Autodesk Fusion 360 part; units mm, degrees
(part 2 of 2)
  spline S76 degree 3 poles (-2.9132, -32.2574) (-2.9111, -32.1274) (-2.9075, -31.9972) (-2.9143, -31.8673) knots 0.000001 0.000001 0.000001 0.000001 1 1 1 1
  line L299 (-5.3918, -31.3025) -> (-5.3918, -30.7233)
  spline S77 degree 3 poles (3.2504, -31.7458) (3.2427, -31.2495) (3.2469, -30.7533) (3.249, -30.2573) knots 0 0 0 0 1 1 1 1
  spline S78 degree 3 poles (0.6248, -32.344) (0.4977, -32.344) (0.3707, -32.3426) (0.2432, -32.3447) knots 0.000001 0.000001 0.000001 0.000001 1 1 1 1
  line L300 (-9.9932, -29.679) -> (-9.9932, -31.7523)
  line L301 (-10.3578, -35.4986) -> (-10.0851, -35.4986)
  line L302 (3.8488, -30.2579) -> (3.8488, -31.7442)
  line L303 (-3.3074, -29.6804) -> (-3.3074, -32.3358)
  spline S79 degree 3 poles (-11.6128, -31.7979) (-11.6121, -31.7822) (-11.5583, -31.7551) (-11.5287, -31.7548) knots 0.000023 0.000023 0.000023 0.000023 1 1 1 1
  line L304 (2.2703, -31.4488) -> (2.2703, -29.6811)
  line L305 (-8.2179, -31.1386) -> (-8.2179, -31.7452)
  spline S80 degree 3 poles (3.249, -30.2573) (3.2504, -29.8676) (3.5651, -29.651) (3.862, -29.6709) knots 0 0 0 0 1 1 1 1
  line L306 (-6.7175, -30.5364) -> (-6.7175, -29.6794)
  line L307 (-8.2179, -31.7452) -> (-6.7246, -31.7452)
  line L308 (-9.9932, -31.7523) -> (-9.8717, -31.7523)
  spline S81 degree 3 poles (0.8918, -30.7238) (0.8571, -30.6827) (0.8217, -30.6427) (0.7622, -30.6077) (0.7622, -30.6076) (0.7621, -30.6076) (0.7621, -30.6076) knots 0 0 0 0 1 1 1 1.000845 1.000845 1.000845 1.000845
  spline S82 degree 3 poles (-0.9957, -31.7527) (-0.8318, -31.7527) (-0.8194, -31.7402) (-0.819, -31.5777) knots 0 0 0 0 1 1 1 1
  spline S83 degree 3 poles (2.1795, -31.3466) (2.2021, -31.3735) (2.2265, -31.3994) (2.2701, -31.4486) (2.2701, -31.4486) (2.2702, -31.4487) (2.2703, -31.4488) knots 0.000001 0.000001 0.000001 0.000001 1 1 1 1.001339 1.001339 1.001339 1.001339
  spline S84 degree 3 poles (-8.2309, -30.5512) (-7.7601, -30.5491) (-7.2897, -30.5459) (-6.8189, -30.5427) knots 0 0 0 0 1 1 1 1
  spline S85 degree 3 poles (-11.6167, -32.3309) (-11.6167, -32.1568) (-11.6188, -31.9773) (-11.6128, -31.7979) knots 0.000143 0.000143 0.000143 0.000143 1 1 1 1
  line L309 (-5.7649, -32.3358) -> (-5.7649, -31.7594)
  line L310 (-5.7639, -30.2551) -> (-5.7639, -29.6804)
  spline S86 degree 3 poles (-10.6833, -31.7527) (-10.6472, -31.7527) (-10.6111, -31.7495) (-10.5669, -31.747) (-10.5668, -31.747) (-10.5668, -31.747) (-10.5668, -31.747) knots 0.000001 0.000001 0.000001 0.000001 1 1 1 1.000711 1.000711 1.000711 1.000711
  line L311 (-6.7246, -31.1386) -> (-8.2179, -31.1386)
  spline S87 degree 3 poles (2.846, -32.3433) (2.6556, -32.3433) (2.4684, -32.3457) (2.2808, -32.3404) knots 0.000175 0.000175 0.000175 0.000175 1 1 1 1
  spline S88 degree 3 poles (-6.2574, -32.3358) (-6.907, -32.3358) (-7.5566, -32.3362) (-8.2061, -32.3358) knots 0 0 0 0 1 1 1 1
  spline S89 degree 3 poles (0.1693, -32.2743) (0.1711, -31.4188) (0.1715, -30.5632) (0.1725, -29.7076) knots 0 0 0 0 1 1 1 1
  spline S90 degree 3 poles (0.1845, -29.6744) (0.3647, -29.6744) (0.5431, -29.6705) (0.7211, -29.6776) knots 0.000128 0.000128 0.000128 0.000128 1 1 1 1
  spline S91 degree 3 poles (-0.8212, -29.6744) (-0.4737, -29.6744) (-0.2415, -29.9051) (-0.2408, -30.2531) knots 0 0 0 0 1 1 1 1
  line L312 (-6.7246, -31.7452) -> (-6.7246, -31.1386)
  spline S92 degree 3 poles (0.2432, -32.3447) (0.1916, -32.3454) (0.169, -32.3285) (0.1693, -32.2743) knots 0.000002 0.000002 0.000002 0.000002 1 1 1 1
  line L313 (6.3064, -30.2505) -> (6.3064, -29.6793)
  line L314 (-5.7649, -31.7594) -> (-3.8959, -31.7594)
  spline S93 degree 3 poles (-8.2061, -32.3358) (-8.5827, -32.3358) (-8.8163, -32.1023) (-8.8167, -31.7271) knots 0 0 0 0 1 1 1 1
  spline S94 degree 3 poles (-5.5311, -34.2712) (-5.5042, -34.6089) (-5.6574, -34.7776) (-5.9909, -34.7776) knots 0 0 0 0 1 1 1 1
  line L315 (-3.8959, -31.3025) -> (-5.3918, -31.3025)
  line L316 (-3.8959, -31.7594) -> (-3.8959, -31.3025)
  spline S95 degree 3 poles (3.862, -29.6709) (4.1049, -29.6868) (4.3498, -29.674) (4.5937, -29.674) knots 0 0 0 0 1 1 1 1
  line L317 (-3.8959, -30.2551) -> (-5.7639, -30.2551)
  spline S96 degree 3 poles (-11.707, -34.2199) (-11.6772, -33.5339) (-11.1336, -33.0249) (-10.4363, -33.0235) knots 0 0 0 0 1 1 1 1
  line L318 (-3.8959, -30.7233) -> (-3.8959, -30.2551)
  spline S97 degree 3 poles (-4.4917, -39.2977) (-4.5365, -39.296) (-4.612, -39.1654) (-4.6134, -39.0936) knots 0 0 0 0 1 1 1 1
  line L319 (-10.3578, -34.3815) -> (-10.3578, -35.4986)
  line L320 (-6.5701, -36.8485) -> (-10.1266, -36.8485)
  spline S98 degree 3 poles (-4.6191, -37.5707) (-4.6191, -36.5314) (-4.6223, -35.4917) (-4.618, -34.4524) knots 0 0 0 0 1 1 1 1
  line L321 (-6.5701, -35.8185) -> (-6.5701, -36.8485)
  line L322 (-2.7841, -30.2505) -> (-2.9061, -30.2505)
  line L323 (-0.819, -31.5777) -> (-0.819, -30.4279)
  line L324 (-5.3918, -30.7233) -> (-3.8959, -30.7233)
  spline S99 degree 3 poles (-6.6217, -34.7812) (-6.8333, -34.7978) (-6.9271, -34.7275) (-6.8956, -34.5116) knots 0 0 0 0 1 1 1 1
  line L325 (-10.1266, -37.9379) -> (-6.9307, -37.9379)
  spline S100 degree 3 poles (-4.6134, -39.0936) (-4.624, -38.5863) (-4.6191, -38.0783) (-4.6191, -37.5707) knots 0 0 0 0 1 1 1 1
  line L326 (-5.7639, -29.6804) -> (-3.3074, -29.6804)
  spline S101 degree 3 poles (0.7211, -29.6776) (0.7571, -29.679) (0.8, -29.7137) (0.8262, -29.7445) knots 0 0 0 0 1 1 1 1
  spline S102 degree 3 poles (-6.8956, -34.5116) (-6.8902, -34.474) (-6.9005, -34.4344) (-6.9051, -34.3816) (-6.9051, -34.3816) (-6.9051, -34.3816) (-6.9051, -34.3815) knots 0 0 0 0 1 1 1 1.000577 1.000577 1.000577 1.000577
  line L327 (2.2703, -29.6811) -> (2.846, -29.6811)
  spline S103 degree 3 poles (-11.7222, -35.3555) (-11.7151, -34.977) (-11.7236, -34.5979) (-11.707, -34.2199) knots 0 0 0 0 1 1 1 1
  line L328 (-6.9051, -34.3815) -> (-10.3578, -34.3815)
  spline S104 degree 3 poles (-11.4978, -36.303) (-11.6914, -36.0138) (-11.7282, -35.691) (-11.7222, -35.3555) knots 0 0 0 0 1 1 1 1
  spline S105 degree 3 poles (1.6966, -39.067) (1.6977, -39.2585) (1.6446, -39.3225) (1.4514, -39.3126) knots 0 0 0 0 1 1 1 1
  spline S106 degree 3 poles (5.3771, -29.674) (5.6864, -29.6758) (5.9253, -29.9126) (5.926, -30.2198) knots 0 0 0 0 1 1 1 1
  spline S107 degree 3 poles (2.7764, -33.7037) (2.5722, -33.4637) (2.5556, -33.3859) (2.6327, -33.0238) knots 0 0 0 0 0.999927 0.999927 0.999927 0.999927
  spline S108 degree 3 poles (3.9383, -35.0656) (3.9383, -35.0656) (3.9383, -35.0655) (3.9382, -35.0655) (3.5287, -34.5855) (3.152, -34.1448) (2.7764, -33.7037) knots -0.000095 -0.000095 -0.000095 -0.000095 0 0 0 1 1 1 1
  line L329 (5.3475, -31.7442) -> (5.3475, -30.2579)
  spline S109 degree 3 poles (1.6916, -34.3533) (1.6938, -35.9247) (1.6888, -37.496) (1.6966, -39.067) knots 0 0 0 0 1 1 1 1
  spline S110 degree 3 poles (5.9303, -31.7596) (5.9374, -32.0226) (5.7452, -32.3365) (5.3683, -32.3415) knots 0 0 0 0 1 1 1 1
  spline S111 degree 3 poles (2.2047, -32.2792) (1.7665, -31.761) (1.3293, -31.2424) (0.8918, -30.7238) knots 0 0 0 0 1 1 1 1
  spline S112 degree 3 poles (5.926, -30.2198) (5.9275, -30.7331) (5.9168, -31.2467) (5.9303, -31.7596) knots 0 0 0 0 1 1 1 1
  spline S113 degree 3 poles (6.299, -32.2566) (6.3018, -32.1232) (6.3032, -31.9897) (6.2983, -31.8563) knots 0 0 0 0 1 1 1 1
  spline S114 degree 3 poles (2.5779, -37.8426) (2.5779, -37.3672) (2.5729, -36.8918) (2.5789, -36.4164) knots 0 0 0 0 1 1 1 1
  line L330 (-3.3074, -32.3358) -> (-5.7649, -32.3358)
  spline S115 degree 3 poles (-3.5897, -33.0536) (-3.4967, -33.0316) (-3.3979, -33.0249) (-3.3016, -33.0249) knots 0 0 0 0 1 1 1 1
  line L331 (-3.2316, -34.3953) -> (-3.2316, -39.3069)
  spline S116 degree 3 poles (8.3973, -29.6748) (8.7371, -29.6748) (8.9753, -29.9087) (8.9767, -30.2467) knots 0 0 0 0 1 1 1 1
  spline S117 degree 3 poles (8.2179, -31.753) (8.385, -31.753) (8.3971, -31.7409) (8.3971, -31.5699) knots 0 0 0 0 1 1 1 1
  spline S118 degree 3 poles (6.4185, -29.6748) (7.078, -29.6748) (7.7375, -29.674) (8.3973, -29.6748) knots 0 0 0 0 1 1 1 1
  spline S119 degree 3 poles (3.7746, -35.0911) (3.8121, -35.0865) (3.8497, -35.0794) (3.9382, -35.0656) (3.9382, -35.0656) (3.9383, -35.0656) (3.9383, -35.0656) knots 0 0 0 0 1 1 1 1.000666 1.000666 1.000666 1.000666
  spline S120 degree 3 poles (0.8262, -29.7445) (1.2786, -30.2772) (1.7285, -30.8121) (2.1795, -31.3466) knots 0 0 0 0 1 1 1 1
  line L332 (-6.4571, -37.4735) -> (-5.5686, -37.4735)
  spline S121 degree 3 poles (3.9098, -33.0302) (3.9802, -33.0323) (4.063, -33.1052) (4.1154, -33.1661) knots 0 0 0 0 1 1 1 1
  spline S122 degree 3 poles (-3.2316, -39.3069) (-3.6723, -39.3069) (-4.0826, -39.3137) (-4.4917, -39.2977) knots 0.000076 0.000076 0.000076 0.000076 1 1 1 1
  line L333 (-10.5668, -31.747) -> (-10.5668, -29.679)
  line L334 (2.846, -29.6811) -> (2.846, -32.3433)
  spline S123 degree 3 poles (-0.819, -30.4279) (-0.819, -30.2793) (-0.8481, -30.2505) (-1.0011, -30.2505) knots 0 0 0 0 1 1 1 1
  spline S124 degree 3 poles (-9.0129, -32.3443) (-9.8685, -32.3426) (-10.7241, -32.3426) (-11.5796, -32.3419) knots 0 0 0 0 1 1 1 1
  spline S125 degree 3 poles (-8.9386, -32.2623) (-8.9379, -32.3154) (-8.951, -32.3443) (-9.0129, -32.3443) knots 0 0 0 0 1 1 1 1
  spline S126 degree 3 poles (-0.2408, -31.7515) (-0.2411, -32.0973) (-0.4556, -32.3355) (-0.8035, -32.3404) knots 0 0 0 0 1 1 1 1
  spline S127 degree 3 poles (-11.5796, -32.3419) (-11.586, -32.3419) (-11.5927, -32.338) (-11.6167, -32.3309) knots 0 0 0 0 0.999006 0.999006 0.999006 0.999006
  spline S128 degree 3 poles (-8.8167, -31.7271) (-8.8167, -31.5285) (-8.8181, -31.3299) (-8.8167, -31.1313) knots 0 0 0 0 1 1 1 1
  spline S129 degree 3 poles (-9.8717, -31.7523) (-9.5934, -31.7523) (-9.3148, -31.7548) (-9.0366, -31.7509) knots 0 0 0 0 1 1 1 1
  line L335 (0.7621, -30.6076) -> (0.7621, -30.7125)
  spline S130 degree 3 poles (-8.9376, -31.8517) (-8.9425, -31.9883) (-8.9401, -32.1253) (-8.9386, -32.2623) knots 0 0 0 0 1 1 1 1
  line L336 (-10.5668, -29.679) -> (-9.9932, -29.679)
  spline S131 degree 3 poles (-9.0366, -31.7509) (-8.9584, -31.7498) (-8.9347, -31.7763) (-8.9376, -31.8517) knots 0 0 0 0 1 1 1 1
  line L337 (7.5171, -33.043) -> (8.8716, -33.043)
  line L338 (7.5171, -35.0688) -> (7.5171, -33.043)
  spline S132 degree 3 poles (0.3636, -33.0242) (1.1324, -33.0253) (1.6906, -33.5831) (1.6916, -34.3533) knots 0 0 0 0 1 1 1 1
  spline S133 degree 3 poles (-5.9909, -34.7776) (-6.2011, -34.7776) (-6.4125, -34.7649) (-6.6217, -34.7812) knots 0 0 0 0 1 1 1 1
  spline S134 degree 3 poles (8.3971, -30.4205) (8.3971, -30.2838) (8.3651, -30.2516) (8.2267, -30.2512) knots 0 0 0 0 1 1 1 1
  spline S135 degree 3 poles (6.404, -31.7512) (7.0086, -31.7544) (7.6133, -31.753) (8.2179, -31.753) knots 0 0 0 0 1 1 1 1
  spline S136 degree 3 poles (2.5789, -36.4164) (2.5878, -35.712) (3.0745, -35.1768) (3.7746, -35.0911) knots 0 0 0 0 1 1 1 1
  spline S137 degree 3 poles (-0.8035, -32.3404) (-1.48, -32.3504) (-2.1572, -32.3429) (-2.834, -32.345) knots 0 0 0 0 1 1 1 1
  spline S138 degree 3 poles (-2.7993, -31.7505) (-2.1982, -31.7544) (-1.5968, -31.7527) (-0.9957, -31.7527) knots 0 0 0 0 1 1 1 1
  spline S139 degree 3 poles (0.5781, -39.3126) (0.3859, -39.3225) (0.3297, -39.2603) (0.3308, -39.0684) knots 0 0 0 0 1 1 1 1
  spline S140 degree 3 poles (-6.8921, -33.0228) (-6.118, -33.0231) (-5.5917, -33.5066) (-5.5311, -34.2712) knots 0 0 0 0 1 1 1 1
  spline S141 degree 3 poles (8.9767, -30.2467) (8.9785, -30.7462) (8.9778, -31.2457) (8.9771, -31.7451) knots 0 0 0 0 1 1 1 1
  spline S142 degree 3 poles (0.3308, -39.0684) (0.3382, -37.5937) (0.3347, -36.1194) (0.3347, -34.6446) knots 0 0 0 0 1 1 1 1
  line L339 (0.3347, -34.6446) -> (0.3346, -34.3953)
  line L340 (3.9933, -36.475) -> (3.9933, -37.8951)
  spline S143 degree 3 poles (2.6327, -33.0238) (3.0554, -33.0238) (3.4829, -33.0175) (3.9098, -33.0302) knots 0.000064 0.000064 0.000064 0.000064 1 1 1 1
  spline S144 degree 3 poles (1.4514, -39.3126) (1.1608, -39.2981) (0.8684, -39.2977) (0.5781, -39.3126) knots 0 0 0 0 1 1 1 1
  line L341 (6.4334, -30.2512) -> (6.3064, -30.2505)
  spline S145 degree 3 poles (-1.0011, -30.2505) (-1.5954, -30.2501) (-2.1897, -30.2505) (-2.7841, -30.2505) knots 0 0 0 0 1 1 1 1
  spline S146 degree 3 poles (8.9771, -31.7451) (8.9767, -32.1023) (8.7474, -32.3404) (8.3871, -32.3429) knots 0 0 0 0 1 1 1 1
  spline S147 degree 3 poles (-5.5686, -37.4735) (-5.351, -38.6001) (-5.9598, -39.3073) (-6.9261, -39.3083) knots 0.000024 0.000024 0.000024 0.000024 1 1 1 1
  spline S148 degree 3 poles (-4.618, -34.4524) (-4.6148, -33.7243) (-4.2297, -33.204) (-3.5897, -33.0536) knots 0 0 0 0 1 1 1 1
  spline S149 degree 3 poles (4.0235, -39.2896) (3.1184, -39.2889) (2.5786, -38.7473) (2.5779, -37.8426) knots 0 0 0 0 1 1 1 1
  spline S150 degree 3 poles (5.5898, -34.8982) (5.667, -34.9863) (5.8128, -35.0575) (5.9297, -35.0614) knots 0 0 0 0 1 1 1 1
  line L342 (3.8488, -31.7442) -> (5.3475, -31.7442)
  spline S151 degree 3 poles (5.9297, -35.0614) (6.4522, -35.0787) (6.9757, -35.0688) (7.517, -35.0688) (7.517, -35.0688) (7.517, -35.0688) (7.5171, -35.0688) knots 0 0 0 0 1 1 1 1.000062 1.000062 1.000062 1.000062
  line L343 (7.5185, -37.8951) -> (7.5185, -36.475)
  line L344 (8.8716, -39.2896) -> (8.586, -39.2896)
  line L345 (8.8716, -33.043) -> (8.8716, -39.2896)
  constraint coincident L131.start L158.end
  constraint midpoint L282 L283.start
emboss "Gravure en relief3" depth 0.3 profiles "Esquisse9" section 1 contours L0 L4 L71 L97 L110 L134 L146 L162 L198 L199 L201 L209 L217 L223 L224 L260 | L1 L2 L109 L113 L169 L174 L175 L179 L184 L185 L186 L203 L212 L219 L259 L267 | L3 L170 L171 L173 L180 L181 L182 L187 L196 L231 L234 L235 L244 L247 L258 L269 L272 L273 L278 L279 | L73 L76 L79 L82 L83 L87 L88 L89 L91 L92 L93 L95 L100 L101 L104 L105 L111 L114 L116 L120 L126 L133 L136 L142 L155 L161 L164 L192 L193 L197 L202 L206 L211 L214 L220 L221 L226 L230 L233 L237 L238 L241 L250 L252 L256 L264 L265 L271 | L74 L90 L123 L125 L128 L147 L188 L228 L232 L239 L245 L248 L251 L253 L262 L268 | L77 L84 L94 L102 L117 L191 L205 L254 | L78 L119 L122 L131 L141 L144 L153 L158 | L172 L176 L227 L243 L249 L255 L266 L277 | L195 L200 L208 L215 L216 L222 L242 L246 L263 L270 | S48 S49 S69 S77 S80 S95 S106 S110 S112 | S50 S57 S107 S108 S114 S119 S121 L337 L338 S136 S143 S149 S150 S151 L344 L345 | S51 L290 S97 S98 S100 S105 S109 S115 L331 S122 S132 S139 S142 L339 S144 S148 | S52 S53 S54 L288 S55 S56 L313 S113 S116 S117 S118 S134 S135 S141 L341 S146 | L289 L291 S60 S72 L296 S75 S76 S82 S91 L322 L323 S123 S126 S137 S138 S145 | S58 S59 L292 S61 S62 S68 S71 L294 S73 S74 L301 S94 S96 L319 L320 L321 S99 L325 S102 S103 L328 S104 L332 S133 S140 S147 | S63 S65 S70 L298 S78 L304 S81 S83 S87 S89 S90 S92 S101 L327 S111 S120 L334 L335 | S64 S67 L293 L295 L297 L306 S84 S88 S93 S128 | S66 L300 S79 L308 S85 S86 L333 S124 S125 S127 S129 S130 L336 S131 | L299 L303 L309 L310 L314 L315 L316 L317 L318 L324 L326 L330 onto face at (14.9255, -36.5, -101.4935) on bodies 7 bodies 7
pattern_circular "Réseau C1" count 3 over 360 about axis through (0, -41, -100) along (0, 1, 0) of "Gravure en relief3"
sketch "Esquisse10" plane through (0, -27.5, 0) normal (0, 1, 0) x (-1, 0, 0)
  circle A0 centre (0, -100) radius 15
  circle A1 centre (0, -100) radius 4.75
  dimension "d121" = 9.5
  constraint concentric A0 A1
  measures "d121" diameter of A1
extrude "Extrusion20" cut sketch "Esquisse10" against normal blind 8.5 contours A1 bodies 7
chamfer "Chanfrein2" distance 0.5 angle 45 1 edges at (-13.9849, -27.5, -94.5758) on bodies 7
fillet "Congé9" radius 0.5 1 edges at (4.4286, -27.5, -98.2823) on bodies 7
hidden bodies 1 2 5 6
